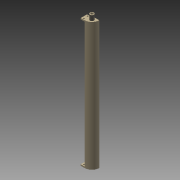
# Autodesk Inventor part: 分离水箱
Saved by Autodesk Inventor 2015 (Build 190159000, 159)
## iProperties
Created: 2017-05-22
Part Number: 分离水箱
Material: 常规
Document SubType Name: Modeling
Designer: Administrator
Density: 1 g/cm^3
Appearance: 米色
Author: Administrator
Autodesk Inventor part; units mm, degrees
ref_plane "YZ Plane" through (0, 0, 0) normal (1, 0, 0) x (0, 1, 0)
ref_plane "XZ Plane" through (0, 0, 0) normal (0, 1, 0) x (-1, 0, 0)
ref_plane "XY Plane" through (0, 0, 0) normal (0, 0, 1) x (1, 0, 0)
sketch "草图1" plane through (0, 0, 0) normal (0, 0, 1) x (1, 0, 0)
  arc A0 (0, -28) -> (28, 0) centre (0, 0) ccw
  line L0 (0, 0) -> (28, 0)
  line L1 (0, 0) -> (0, -28)
  dimension "d0" = 28
  constraints: 4 end point, 2 point on circle, 1 centre point, 1 coincident, 1 horizontal, 1 vertical
  measures "d0" radius of A0
extrude "拉伸1" add sketch "草图1" along normal blind 480
shell "抽壳1" thickness 2 removed faces 1 at (13.1163, -13.1163, 480)
sketch "草图2" plane through (0, 0, 480) normal (0, 0, 1) x (1, 0, 0)
  line L0 (0, -28) -> (-15, -28)
  line L1 (-15, -28) -> (-15, 0)
  line L2 (-15, 0) -> (0, 0)
  line L3 (0, 0) -> (0, -28)
  line L4 (28, 0) -> (0, 0) projected
  arc A0 (0, -28) -> (28, 0) centre (0, 0) ccw
  line L5 (0, 0) -> (28, 0)
  line L6 (0, 0) -> (0, -28)
  line L7 (0, 0) -> (0, -28) projected
  dimension "d4" = 15
  constraints: 12 end point, 4 equal length, 2 point on circle, 1 centre point, 1 collinear, 1 horizontal, 1 perpendicular, 1 tangent
  measures "d4" distance of L1.end L2.end
extrude "拉伸2" add sketch "草图2" along normal blind 5
sketch "草图3" plane through (0, 0, 485) normal (0, 0, 1) x (1, 0, 0)
  circle A0 centre (11.598, -11.598) radius 7.5
  circle A1 centre (11.598, -11.598) radius 11.598
  line L0 (28, 0) -> (-15, 0) projected
  line L1 (0, 0) -> (0, -28) projected
  arc A2 (0, -28) -> (28, 0) centre (0, 0) ccw projected
  dimension "d7" = 15
  constraints: 3 tangent, 2 centre point, 1 coincident
  measures "d7" diameter of A0
extrude "拉伸3" add sketch "草图3" along normal blind 20 contours A0
sketch "草图4" plane through (11.598, -11.598, 505) normal (0, 0, 1) x (1, 0, 0)
  circle A0 centre (0, 0) radius 5
  circle A1 centre (0, 0) radius 7.5 projected
  point P0 (-11.598, 11.598)
  dimension "d10" = 10
  constraints: 1 centre point, 1 concentric
  measures "d10" diameter of A0
extrude "拉伸4" cut sketch "草图4" against normal up to surface (25 mm away) contours A0
thread "螺纹1" size "M15x1.5" class "6g" standard "ANSI Metric M Profile" full length
chamfer "倒角1" distance 0.5 angle 45 1 edges at (4.098, -11.598, 505)
sketch "草图5" plane through (0, 0, 0) normal (0, 0, -1) x (-1, 0, 0)
  arc A0 (-28, 0) -> (0, -28) centre (0, 0) ccw
  line L0 (-28, 0) -> (15, 0)
  line L1 (-28, 0) -> (15, 0) projected
  line L2 (15, 0) -> (15, -28)
  line L3 (15, 0) -> (15, -28) projected
  line L4 (15, -28) -> (0, -28)
  line L5 (15, -28) -> (0, -28) projected
  arc A1 (-25.923, -2) -> (-2, -25.923) centre (0, 0) ccw projected
  constraints: 6 end point, 3 collinear, 2 point on circle, 1 centre point, 1 concentric
extrude "拉伸5" add sketch "草图5" along normal blind 5
sketch "草图6" plane through (0, 0, 485) normal (0, 0, 1) x (1, 0, 0)
  circle A0 centre (-7.5, -9) radius 2.5
  circle A1 centre (-7.5, -23) radius 2.5
  line L0 (28, 0) -> (-15, 0) projected
  line L1 (-15, -28) -> (0, -28) projected
  line L2 (-15, 0) -> (-15, -28) projected
  point P0 (0, 0)
  dimension "d20" = 5
  dimension "d21" = 5
  dimension "d22" = 9
  dimension "d23" = 5
  dimension "d24" = 7.5
  dimension "d25" = 7.5
  constraints: 2 centre point
  measures "d20" diameter of A0
  measures "d21" diameter of A1
  measures "d22" distance from line of L0 A0.centre
  measures "d23" distance from line of L1 A1.centre
  measures "d24" distance from line of L2 A0.centre
  measures "d25" distance from line of L2 A1.centre
extrude "拉伸6" cut sketch "草图6" against normal through all
sketch "草图7" plane through (0, 0, 485) normal (0, 0, 1) x (1, 0, 0)
  line L0 (-15, 0) -> (0, 0)
  line L1 (0, 0) -> (0, -4)
  line L2 (0, -4) -> (-15, -4)
  line L3 (-15, -4) -> (-15, 0)
  line L4 (0, 0) -> (0, -28) projected
  line L5 (28, 0) -> (-15, 0) projected
  line L6 (-15, 0) -> (-15, -28) projected
  dimension "d28" = 4
  constraints: 8 end point, 3 collinear, 2 parallel, 1 horizontal, 1 perpendicular
  measures "d28" distance between parallel lines of L0 L2
extrude "拉伸7" cut sketch "草图7" against normal through all
sketch "草图8" plane through (0, 0, -5) normal (-1, 0, 0) x (0, 0, 1)
  line L0 (7, -25.923) -> (485, -25.923) projected
  line L1 (470, -25.923) -> (450, -25.923)
  line L2 (450, -25.923) -> (450, -23.923)
  line L3 (450, -23.923) -> (470, -23.923)
  line L4 (470, -23.923) -> (470, -25.923)
  line L5 (485, -4) -> (485, -28) projected
  point P0 (5, 0)
  dimension "d31" = 20
  dimension "d32" = 2
  dimension "d33" = 15
  constraints: 8 end point, 2 parallel, 1 horizontal, 1 perpendicular, 1 point on line
  measures "d31" distance of L2.end L3.end
  measures "d32" distance of L1.end L2.end
  measures "d33" distance between parallel lines of L5 L4
extrude "拉伸8" cut sketch "草图8" against normal blind 2
pattern_linear "矩形阵列1" count 2 spacing 70 along (0, 0, -1) of "拉伸8"
pattern_linear "矩形阵列2" count 4 spacing 120 along (0, 0, -1) of "拉伸8", "矩形阵列1"
